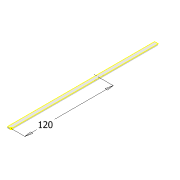
# Autodesk Inventor part: Feather_0_aerofoil_frame_support
Saved by Autodesk Inventor 2022 (Build 260153000, 153)
## iProperties
Created: 2022-09-01
Part Number: Feather_0_aerofoil_frame_support
Material: Generic
Document SubType Name: Modeling
Designer: dell
Density: 1 g/cm^3
Appearance: Default
Author: dell
Autodesk Inventor part; units mm, degrees
ref_plane "YZ Plane" through (0, 0, 0) normal (1, 0, 0) x (0, 1, 0)
ref_plane "XZ Plane" through (0, 0, 0) normal (0, 1, 0) x (-1, 0, 0)
ref_plane "XY Plane" through (0, 0, 0) normal (0, 0, 1) x (1, 0, 0)
sketch "Sketch1" plane through (0, 0, 0) normal (0, 1, 0) x (-1, 0, 0)
  line L0 (0, 0) -> (5, 0)
  line L1 (5, 0) -> (5, -200)
  line L2 (5, -200) -> (0, -200)
  line L3 (0, -200) -> (0, 0)
  dimension "d0" = 5
  dimension "d1" = 200
  constraints: 8 end point, 2 parallel, 1 horizontal, 1 perpendicular
  measures "d0" distance of L0.start L0.end
  measures "d1" distance between parallel lines of L2 L0
extrude "Extrusion1" add sketch "Sketch1" along normal blind 2
sketch "Sketch2" plane through (0, 2, 0) normal (0, 1, 0) x (1, 0, 0)
  line L0 (0, 200) -> (-5, 200) projected
  line L1 (-5, 200) -> (-5, 0) projected
  line L2 (-5, 0) -> (0, 0) projected
  line L3 (0, 0) -> (0, 200) projected
sketch "Sketch3" plane through (0, 2, 0) normal (0, 1, 0) x (1, 0, 0)
  line L0 (0, 0) -> (0, 200) projected
  point P0 (0, 120)
  dimension "d4" = 120
  constraints: 1 point on line
  measures "d4" distance of L0.start point (0, 120)
body "Solid1"
